Autodesk Fusion 360 part; units mm, degrees
(part 2 of 5)
ref_plane "工作平面7" through (0, 0, 26) normal (0, 0, 1) x (1, 0, 0) in component "L2_RemovableGrate"
sketch "草图7 (6)" plane through (0, 0, 26) normal (0, 0, 1) x (1, 0, 0) in component "L2_RemovableGrate"
  line L0 (299, 60.3) -> (303, 60.3)
  line L1 (303, 60.3) -> (303, 129.7)
  line L2 (303, 129.7) -> (299, 129.7)
  line L3 (299, 129.7) -> (299, 60.3)
  dimension "d537" = 299
  dimension "d539" = 4
  dimension "d540" = 69.4
  constraint horizontal L0
  constraint vertical L1
  constraint horizontal L2
  constraint vertical L3
  measures "d537" horizontal distance of origin L0.start
  measures "d539" horizontal distance of L0.start L0.end
  measures "d540" vertical distance of L0.end L1.end
extrude "Drain slot 6''" cut sketch "草图7 (6)" along normal blind 4 bodies 6 in component "L2_RemovableGrate"
ref_plane "工作平面8" through (0, 0, 26) normal (0, 0, 1) x (1, 0, 0) in component "L2_RemovableGrate"
sketch "草图8 (6)" plane through (0, 0, 26) normal (0, 0, 1) x (1, 0, 0) in component "L2_RemovableGrate"
  line L0 (309, 60.3) -> (313, 60.3)
  line L1 (313, 60.3) -> (313, 129.7)
  line L2 (313, 129.7) -> (309, 129.7)
  line L3 (309, 129.7) -> (309, 60.3)
  dimension "d545" = 309
  dimension "d547" = 4
  dimension "d548" = 69.4
  constraint horizontal L0
  constraint vertical L1
  constraint horizontal L2
  constraint vertical L3
  measures "d545" horizontal distance of origin L0.start
  measures "d547" horizontal distance of L0.start L0.end
  measures "d548" vertical distance of L0.end L1.end
extrude "Drain slot 7''" cut sketch "草图8 (6)" along normal blind 4 bodies 6 in component "L2_RemovableGrate"
ref_plane "工作平面9" through (0, 0, 26) normal (0, 0, 1) x (1, 0, 0) in component "L2_RemovableGrate"
sketch "草图9 (3)" plane through (0, 0, 26) normal (0, 0, 1) x (1, 0, 0) in component "L2_RemovableGrate"
  line L0 (319, 60.3) -> (323, 60.3)
  line L1 (323, 60.3) -> (323, 129.7)
  line L2 (323, 129.7) -> (319, 129.7)
  line L3 (319, 129.7) -> (319, 60.3)
  dimension "d553" = 319
  dimension "d555" = 4
  dimension "d556" = 69.4
  constraint horizontal L0
  constraint vertical L1
  constraint horizontal L2
  constraint vertical L3
  measures "d553" horizontal distance of origin L0.start
  measures "d555" horizontal distance of L0.start L0.end
  measures "d556" vertical distance of L0.end L1.end
extrude "Drain slot 8''" cut sketch "草图9 (3)" along normal blind 4 bodies 6 in component "L2_RemovableGrate"
ref_plane "工作平面10" through (0, 0, 26) normal (0, 0, 1) x (1, 0, 0) in component "L2_RemovableGrate"
sketch "草图10 (3)" plane through (0, 0, 26) normal (0, 0, 1) x (1, 0, 0) in component "L2_RemovableGrate"
  line L0 (329, 60.3) -> (333, 60.3)
  line L1 (333, 60.3) -> (333, 129.7)
  line L2 (333, 129.7) -> (329, 129.7)
  line L3 (329, 129.7) -> (329, 60.3)
  dimension "d561" = 329
  dimension "d563" = 4
  dimension "d564" = 69.4
  constraint horizontal L0
  constraint vertical L1
  constraint horizontal L2
  constraint vertical L3
  measures "d561" horizontal distance of origin L0.start
  measures "d563" horizontal distance of L0.start L0.end
  measures "d564" vertical distance of L0.end L1.end
extrude "Drain slot 9''" cut sketch "草图10 (3)" along normal blind 4 bodies 6 in component "L2_RemovableGrate"
ref_plane "工作平面11" through (0, 0, 26) normal (0, 0, 1) x (1, 0, 0) in component "L2_RemovableGrate"
sketch "草图11 (3)" plane through (0, 0, 26) normal (0, 0, 1) x (1, 0, 0) in component "L2_RemovableGrate"
  line L0 (339, 60.3) -> (343, 60.3)
  line L1 (343, 60.3) -> (343, 129.7)
  line L2 (343, 129.7) -> (339, 129.7)
  line L3 (339, 129.7) -> (339, 60.3)
  dimension "d569" = 339
  dimension "d571" = 4
  dimension "d572" = 69.4
  constraint horizontal L0
  constraint vertical L1
  constraint horizontal L2
  constraint vertical L3
  measures "d569" horizontal distance of origin L0.start
  measures "d571" horizontal distance of L0.start L0.end
  measures "d572" vertical distance of L0.end L1.end
extrude "Drain slot 10''" cut sketch "草图11 (3)" along normal blind 4 bodies 6 in component "L2_RemovableGrate"
ref_plane "工作平面12" through (0, 0, 26) normal (0, 0, 1) x (1, 0, 0) in component "L2_RemovableGrate"
sketch "草图12 (3)" plane through (0, 0, 26) normal (0, 0, 1) x (1, 0, 0) in component "L2_RemovableGrate"
  line L0 (349, 60.3) -> (353, 60.3)
  line L1 (353, 60.3) -> (353, 129.7)
  line L2 (353, 129.7) -> (349, 129.7)
  line L3 (349, 129.7) -> (349, 60.3)
  dimension "d577" = 349
  dimension "d579" = 4
  dimension "d580" = 69.4
  constraint horizontal L0
  constraint vertical L1
  constraint horizontal L2
  constraint vertical L3
  measures "d577" horizontal distance of origin L0.start
  measures "d579" horizontal distance of L0.start L0.end
  measures "d580" vertical distance of L0.end L1.end
extrude "Drain slot 11''" cut sketch "草图12 (3)" along normal blind 4 bodies 6 in component "L2_RemovableGrate"
ref_plane "工作平面13" through (0, 0, 26) normal (0, 0, 1) x (1, 0, 0) in component "L2_RemovableGrate"
sketch "草图13 (3)" plane through (0, 0, 26) normal (0, 0, 1) x (1, 0, 0) in component "L2_RemovableGrate"
  line L0 (359, 60.3) -> (363, 60.3)
  line L1 (363, 60.3) -> (363, 129.7)
  line L2 (363, 129.7) -> (359, 129.7)
  line L3 (359, 129.7) -> (359, 60.3)
  dimension "d585" = 359
  dimension "d587" = 4
  dimension "d588" = 69.4
  constraint horizontal L0
  constraint vertical L1
  constraint horizontal L2
  constraint vertical L3
  measures "d585" horizontal distance of origin L0.start
  measures "d587" horizontal distance of L0.start L0.end
  measures "d588" vertical distance of L0.end L1.end
extrude "Drain slot 12'" cut sketch "草图13 (3)" along normal blind 4 bodies 6 in component "L2_RemovableGrate"
ref_plane "工作平面14" through (0, 0, 26) normal (0, 0, 1) x (1, 0, 0) in component "L2_RemovableGrate"
sketch "草图14 (2)" plane through (0, 0, 26) normal (0, 0, 1) x (1, 0, 0) in component "L2_RemovableGrate"
  line L0 (369, 60.3) -> (373, 60.3)
  line L1 (373, 60.3) -> (373, 129.7)
  line L2 (373, 129.7) -> (369, 129.7)
  line L3 (369, 129.7) -> (369, 60.3)
  dimension "d593" = 369
  dimension "d595" = 4
  dimension "d596" = 69.4
  constraint horizontal L0
  constraint vertical L1
  constraint horizontal L2
  constraint vertical L3
  measures "d593" horizontal distance of origin L0.start
  measures "d595" horizontal distance of L0.start L0.end
  measures "d596" vertical distance of L0.end L1.end
extrude "Drain slot 13'" cut sketch "草图14 (2)" along normal blind 4 bodies 6 in component "L2_RemovableGrate"
ref_plane "工作平面15" through (0, 0, 26) normal (0, 0, 1) x (1, 0, 0) in component "L2_RemovableGrate"
sketch "草图15 (2)" plane through (0, 0, 26) normal (0, 0, 1) x (1, 0, 0) in component "L2_RemovableGrate"
  line L0 (379, 60.3) -> (383, 60.3)
  line L1 (383, 60.3) -> (383, 129.7)
  line L2 (383, 129.7) -> (379, 129.7)
  line L3 (379, 129.7) -> (379, 60.3)
  dimension "d601" = 379
  dimension "d603" = 4
  dimension "d604" = 69.4
  constraint horizontal L0
  constraint vertical L1
  constraint horizontal L2
  constraint vertical L3
  measures "d601" horizontal distance of origin L0.start
  measures "d603" horizontal distance of L0.start L0.end
  measures "d604" vertical distance of L0.end L1.end
extrude "Drain slot 14'" cut sketch "草图15 (2)" along normal blind 4 bodies 6 in component "L2_RemovableGrate"
ref_plane "工作平面16" through (0, 0, 26) normal (0, 0, 1) x (1, 0, 0) in component "L2_RemovableGrate"
sketch "草图16 (2)" plane through (0, 0, 26) normal (0, 0, 1) x (1, 0, 0) in component "L2_RemovableGrate"
  line L0 (389, 60.3) -> (393, 60.3)
  line L1 (393, 60.3) -> (393, 129.7)
  line L2 (393, 129.7) -> (389, 129.7)
  line L3 (389, 129.7) -> (389, 60.3)
  dimension "d609" = 389
  dimension "d611" = 4
  dimension "d612" = 69.4
  constraint horizontal L0
  constraint vertical L1
  constraint horizontal L2
  constraint vertical L3
  measures "d609" horizontal distance of origin L0.start
  measures "d611" horizontal distance of L0.start L0.end
  measures "d612" vertical distance of L0.end L1.end
extrude "Drain slot 15'" cut sketch "草图16 (2)" along normal blind 4 bodies 6 in component "L2_RemovableGrate"
ref_plane "工作平面17" through (0, 0, 26) normal (0, 0, 1) x (1, 0, 0) in component "L2_RemovableGrate"
sketch "草图17 (2)" plane through (0, 0, 26) normal (0, 0, 1) x (1, 0, 0) in component "L2_RemovableGrate"
  line L0 (399, 60.3) -> (403, 60.3)
  line L1 (403, 60.3) -> (403, 129.7)
  line L2 (403, 129.7) -> (399, 129.7)
  line L3 (399, 129.7) -> (399, 60.3)
  dimension "d617" = 399
  dimension "d619" = 4
  dimension "d620" = 69.4
  constraint horizontal L0
  constraint vertical L1
  constraint horizontal L2
  constraint vertical L3
  measures "d617" horizontal distance of origin L0.start
  measures "d619" horizontal distance of L0.start L0.end
  measures "d620" vertical distance of L0.end L1.end
extrude "Drain slot 16" cut sketch "草图17 (2)" along normal blind 4 bodies 6 in component "L2_RemovableGrate"
ref_plane "工作平面18" through (0, 0, 26) normal (0, 0, 1) x (1, 0, 0) in component "L2_RemovableGrate"
sketch "草图18" plane through (0, 0, 26) normal (0, 0, 1) x (1, 0, 0) in component "L2_RemovableGrate"
  line L0 (409, 60.3) -> (413, 60.3)
  line L1 (413, 60.3) -> (413, 129.7)
  line L2 (413, 129.7) -> (409, 129.7)
  line L3 (409, 129.7) -> (409, 60.3)
  dimension "d625" = 409
  dimension "d627" = 4
  dimension "d628" = 69.4
  constraint horizontal L0
  constraint vertical L1
  constraint horizontal L2
  constraint vertical L3
  measures "d625" horizontal distance of origin L0.start
  measures "d627" horizontal distance of L0.start L0.end
  measures "d628" vertical distance of L0.end L1.end
extrude "Drain slot 17" cut sketch "草图18" along normal blind 4 bodies 6 in component "L2_RemovableGrate"
ref_plane "工作平面19" through (0, 0, 26) normal (0, 0, 1) x (1, 0, 0) in component "L2_RemovableGrate"
sketch "草图19" plane through (0, 0, 26) normal (0, 0, 1) x (1, 0, 0) in component "L2_RemovableGrate"
  line L0 (323, 132.7) -> (339, 132.7)
  line L1 (339, 132.7) -> (339, 137.7)
  line L2 (339, 137.7) -> (323, 137.7)
  line L3 (323, 137.7) -> (323, 132.7)
  dimension "d633" = 323
  dimension "d634" = 132.7
  dimension "d635" = 16
  dimension "d636" = 5
  constraint horizontal L0
  constraint vertical L1
  constraint horizontal L2
  constraint vertical L3
  measures "d633" horizontal distance of origin L0.start
  measures "d634" vertical distance of origin L0.start
  measures "d635" horizontal distance of L0.start L0.end
  measures "d636" vertical distance of L0.end L1.end
extrude "Finger lift notch''" cut sketch "草图19" along normal blind 4 bodies 6 in component "L2_RemovableGrate"
chamfer "R03 touch edge chamfer'''''" distance 0.4 angle 45 5 edges at (279.15, 136.7, 30) (235.3, 95, 30) (331, 53.3, 30) (426.7, 95, 30) (382.85, 136.7, 30) on bodies 6 in component "L2_RemovableGrate"
ref_plane "工作平面1" through (0, 0, 10) normal (0, 0, 1) x (1, 0, 0) in component "R2_Integrated"
sketch "草图1 (7)" plane through (0, 0, 10) normal (0, 0, 1) x (1, 0, 0) in component "R2_Integrated"
  line L0 (726, 50) -> (860, 50)
  line L1 (860, 50) -> (860, 140)
  line L2 (860, 140) -> (726, 140)
  line L3 (726, 140) -> (726, 50)
  dimension "d642" = 726
  dimension "d643" = 50
  dimension "d644" = 134
  dimension "d645" = 90
  constraint horizontal L0
  constraint vertical L1
  constraint horizontal L2
  constraint vertical L3
  measures "d642" horizontal distance of origin L0.start
  measures "d643" vertical distance of origin L0.start
  measures "d644" horizontal distance of L0.start L0.end
  measures "d645" vertical distance of L0.end L1.end
extrude "R04 pan blank'''" add sketch "草图1 (7)" along normal blind 20 separate body makes body 7 in component "R2_Integrated"
fillet "Outside corner rounds'''" radius 3 4 edges at (726, 140, 20) (860, 140, 20) (860, 50, 20) (726, 50, 20) on bodies 7 in component "R2_Integrated"
ref_plane "工作平面2" through (729, 0, 0) normal (1, 0, 0) x (0, 1, 0) in component "R2_Integrated"
sketch "草图2 (7)" plane through (729, 0, 0) normal (1, 0, 0) x (0, 0, -1) in component "R2_Integrated"
  line L0 (-22.1441, 53) -> (-13, 140)
  line L1 (-13, 140) -> (-31, 140)
  line L2 (-31, 140) -> (-31, 53)
  line L3 (-31, 53) -> (-22.1441, 53)
  dimension "d654" = 13
  dimension "d656" = 31
  constraint horizontal L1
  constraint vertical L2
  constraint horizontal L3
  measures "d654" horizontal distance of origin L0.end
  measures "d656" horizontal distance of origin L1.end
extrude "R04 continuous slope and open edge'''" cut sketch "草图2 (7)" along normal blind 128 bodies 7 in component "R2_Integrated"
ref_plane "工作平面3" through (0, 0, 10) normal (0, 0, 1) x (1, 0, 0) in component "R2_Integrated"
sketch "草图3 (7)" plane through (0, 0, 10) normal (0, 0, 1) x (1, 0, 0) in component "R2_Integrated"
  line L0 (729, 53) -> (741, 53)
  line L1 (741, 53) -> (741, 65)
  line L2 (741, 65) -> (729, 65)
  line L3 (729, 65) -> (729, 53)
  dimension "d661" = 729
  dimension "d663" = 12
  dimension "d664" = 12
  constraint horizontal L0
  constraint vertical L1
  constraint horizontal L2
  constraint vertical L3
  measures "d661" horizontal distance of origin L0.start
  measures "d663" horizontal distance of L0.start L0.end
  measures "d664" vertical distance of L0.end L1.end
extrude "Grate seat 00'''" add sketch "草图3 (7)" along normal blind 16 bodies 7 in component "R2_Integrated"
ref_plane "工作平面4" through (0, 0, 10) normal (0, 0, 1) x (1, 0, 0) in component "R2_Integrated"
sketch "草图4 (7)" plane through (0, 0, 10) normal (0, 0, 1) x (1, 0, 0) in component "R2_Integrated"
  line L0 (729, 125) -> (741, 125)
  line L1 (741, 125) -> (741, 137)
  line L2 (741, 137) -> (729, 137)
  line L3 (729, 137) -> (729, 125)
  dimension "d669" = 729
  dimension "d670" = 125
  dimension "d671" = 12
  dimension "d672" = 12
  constraint horizontal L0
  constraint vertical L1
  constraint horizontal L2
  constraint vertical L3
  measures "d669" horizontal distance of origin L0.start
  measures "d670" vertical distance of origin L0.start
  measures "d671" horizontal distance of L0.start L0.end
  measures "d672" vertical distance of L0.end L1.end
extrude "Grate seat 01'''" add sketch "草图4 (7)" along normal blind 16 bodies 7 in component "R2_Integrated"
ref_plane "工作平面5" through (0, 0, 10) normal (0, 0, 1) x (1, 0, 0) in component "R2_Integrated"
sketch "草图5 (7)" plane through (0, 0, 10) normal (0, 0, 1) x (1, 0, 0) in component "R2_Integrated"
  line L0 (845, 53) -> (857, 53)
  line L1 (857, 53) -> (857, 65)
  line L2 (857, 65) -> (845, 65)
  line L3 (845, 65) -> (845, 53)
  dimension "d677" = 845
  dimension "d679" = 12
  dimension "d680" = 12
  constraint horizontal L0
  constraint vertical L1
  constraint horizontal L2
  constraint vertical L3
  measures "d677" horizontal distance of origin L0.start
  measures "d679" horizontal distance of L0.start L0.end
  measures "d680" vertical distance of L0.end L1.end
extrude "Grate seat 10'''" add sketch "草图5 (7)" along normal blind 16 bodies 7 in component "R2_Integrated"
ref_plane "工作平面6" through (0, 0, 10) normal (0, 0, 1) x (1, 0, 0) in component "R2_Integrated"
sketch "草图6 (7)" plane through (0, 0, 10) normal (0, 0, 1) x (1, 0, 0) in component "R2_Integrated"
  line L0 (845, 125) -> (857, 125)
  line L1 (857, 125) -> (857, 137)
  line L2 (857, 137) -> (845, 137)
  line L3 (845, 137) -> (845, 125)
  dimension "d685" = 845
  dimension "d686" = 125
  dimension "d687" = 12
  dimension "d688" = 12
  constraint horizontal L0
  constraint vertical L1
  constraint horizontal L2
  constraint vertical L3
  measures "d685" horizontal distance of origin L0.start
  measures "d686" vertical distance of origin L0.start
  measures "d687" horizontal distance of L0.start L0.end
  measures "d688" vertical distance of L0.end L1.end
extrude "Grate seat 11'''" add sketch "草图6 (7)" along normal blind 16 bodies 7 in component "R2_Integrated"
ref_plane "工作平面7" through (0, 0, 0) normal (0, 0, 1) x (1, 0, 0) in component "R2_Integrated"
sketch "草图7 (7)" plane through (0, 0, 0) normal (0, 0, 1) x (1, 0, 0) in component "R2_Integrated"
  line L0 (729, 50) -> (737, 50)
  line L1 (737, 50) -> (737, 131)
  line L2 (737, 131) -> (729, 131)
  line L3 (729, 131) -> (729, 50)
  dimension "d693" = 729
  dimension "d694" = 50
  dimension "d695" = 8
  dimension "d696" = 81
  constraint horizontal L0
  constraint vertical L1
  constraint horizontal L2
  constraint vertical L3
  measures "d693" horizontal distance of origin L0.start
  measures "d694" vertical distance of origin L0.start
  measures "d695" horizontal distance of L0.start L0.end
  measures "d696" vertical distance of L0.end L1.end
extrude "R04 low integral runner 0'''" add sketch "草图7 (7)" along normal blind 10 bodies 7 in component "R2_Integrated"
ref_plane "工作平面8" through (0, 0, 0) normal (0, 0, 1) x (1, 0, 0) in component "R2_Integrated"
sketch "草图8 (7)" plane through (0, 0, 0) normal (0, 0, 1) x (1, 0, 0) in component "R2_Integrated"
  line L0 (849, 50) -> (857, 50)
  line L1 (857, 50) -> (857, 131)
  line L2 (857, 131) -> (849, 131)
  line L3 (849, 131) -> (849, 50)
  dimension "d701" = 849
  dimension "d702" = 50
  dimension "d703" = 8
  dimension "d704" = 81
  constraint horizontal L0
  constraint vertical L1
  constraint horizontal L2
  constraint vertical L3
  measures "d701" horizontal distance of origin L0.start
  measures "d702" vertical distance of origin L0.start
  measures "d703" horizontal distance of L0.start L0.end
  measures "d704" vertical distance of L0.end L1.end
extrude "R04 low integral runner 1'''" add sketch "草图8 (7)" along normal blind 10 bodies 7 in component "R2_Integrated"
chamfer "R03 touch edge chamfer''''''" distance 0.4 angle 45 5 edges at (793, 53, 30) (729, 96.5, 30) (857, 96.5, 30) (726, 95, 30) (860, 95, 30) on bodies 7 in component "R2_Integrated"
ref_plane "工作平面1" through (0, 0, 26) normal (0, 0, 1) x (1, 0, 0) in component "R2_RemovableGrate"
sketch "草图1 (8)" plane through (0, 0, 26) normal (0, 0, 1) x (1, 0, 0) in component "R2_RemovableGrate"
  line L0 (729.3, 53.3) -> (856.7, 53.3)
  line L1 (856.7, 53.3) -> (856.7, 136.7)
  line L2 (856.7, 136.7) -> (729.3, 136.7)
  line L3 (729.3, 136.7) -> (729.3, 53.3)
  dimension "d710" = 729.3
  dimension "d712" = 127.4
  dimension "d713" = 83.4
  constraint horizontal L0
  constraint vertical L1
  constraint horizontal L2
  constraint vertical L3
  measures "d710" horizontal distance of origin L0.start
  measures "d712" horizontal distance of L0.start L0.end
  measures "d713" vertical distance of L0.end L1.end
extrude "Horizontal removable deck'''" add sketch "草图1 (8)" along normal blind 4 separate body makes body 8 in component "R2_RemovableGrate"
ref_plane "工作平面2" through (0, 0, 26) normal (0, 0, 1) x (1, 0, 0) in component "R2_RemovableGrate"
sketch "草图2 (8)" plane through (0, 0, 26) normal (0, 0, 1) x (1, 0, 0) in component "R2_RemovableGrate"
  line L0 (741, 60.3) -> (745, 60.3)
  line L1 (745, 60.3) -> (745, 129.7)
  line L2 (745, 129.7) -> (741, 129.7)
  line L3 (741, 129.7) -> (741, 60.3)
  dimension "d718" = 741
  dimension "d720" = 4
  dimension "d721" = 69.4
  constraint horizontal L0
  constraint vertical L1
  constraint horizontal L2
  constraint vertical L3
  measures "d718" horizontal distance of origin L0.start
  measures "d720" horizontal distance of L0.start L0.end
  measures "d721" vertical distance of L0.end L1.end
extrude "Drain slot 1'''" cut sketch "草图2 (8)" along normal blind 4 bodies 8 in component "R2_RemovableGrate"
ref_plane "工作平面3" through (0, 0, 26) normal (0, 0, 1) x (1, 0, 0) in component "R2_RemovableGrate"
sketch "草图3 (8)" plane through (0, 0, 26) normal (0, 0, 1) x (1, 0, 0) in component "R2_RemovableGrate"
  line L0 (751, 60.3) -> (755, 60.3)
  line L1 (755, 60.3) -> (755, 129.7)
  line L2 (755, 129.7) -> (751, 129.7)
  line L3 (751, 129.7) -> (751, 60.3)
  dimension "d726" = 751
  dimension "d728" = 4
  dimension "d729" = 69.4
  constraint horizontal L0
  constraint vertical L1
  constraint horizontal L2
  constraint vertical L3
  measures "d726" horizontal distance of origin L0.start
  measures "d728" horizontal distance of L0.start L0.end
  measures "d729" vertical distance of L0.end L1.end
extrude "Drain slot 2'''" cut sketch "草图3 (8)" along normal blind 4 bodies 8 in component "R2_RemovableGrate"
ref_plane "工作平面4" through (0, 0, 26) normal (0, 0, 1) x (1, 0, 0) in component "R2_RemovableGrate"
sketch "草图4 (8)" plane through (0, 0, 26) normal (0, 0, 1) x (1, 0, 0) in component "R2_RemovableGrate"
  line L0 (761, 60.3) -> (765, 60.3)
  line L1 (765, 60.3) -> (765, 129.7)
  line L2 (765, 129.7) -> (761, 129.7)
  line L3 (761, 129.7) -> (761, 60.3)
  dimension "d734" = 761
  dimension "d736" = 4
  dimension "d737" = 69.4
  constraint horizontal L0
  constraint vertical L1
  constraint horizontal L2
  constraint vertical L3
  measures "d734" horizontal distance of origin L0.start
  measures "d736" horizontal distance of L0.start L0.end
  measures "d737" vertical distance of L0.end L1.end
extrude "Drain slot 3'''" cut sketch "草图4 (8)" along normal blind 4 bodies 8 in component "R2_RemovableGrate"
ref_plane "工作平面5" through (0, 0, 26) normal (0, 0, 1) x (1, 0, 0) in component "R2_RemovableGrate"
sketch "草图5 (8)" plane through (0, 0, 26) normal (0, 0, 1) x (1, 0, 0) in component "R2_RemovableGrate"
  line L0 (771, 60.3) -> (775, 60.3)
  line L1 (775, 60.3) -> (775, 129.7)
  line L2 (775, 129.7) -> (771, 129.7)
  line L3 (771, 129.7) -> (771, 60.3)
  dimension "d742" = 771
  dimension "d744" = 4
  dimension "d745" = 69.4
  constraint horizontal L0
  constraint vertical L1
  constraint horizontal L2
  constraint vertical L3
  measures "d742" horizontal distance of origin L0.start
  measures "d744" horizontal distance of L0.start L0.end
  measures "d745" vertical distance of L0.end L1.end
extrude "Drain slot 4'''" cut sketch "草图5 (8)" along normal blind 4 bodies 8 in component "R2_RemovableGrate"
ref_plane "工作平面6" through (0, 0, 26) normal (0, 0, 1) x (1, 0, 0) in component "R2_RemovableGrate"
sketch "草图6 (8)" plane through (0, 0, 26) normal (0, 0, 1) x (1, 0, 0) in component "R2_RemovableGrate"
  line L0 (781, 60.3) -> (785, 60.3)
  line L1 (785, 60.3) -> (785, 129.7)
  line L2 (785, 129.7) -> (781, 129.7)
  line L3 (781, 129.7) -> (781, 60.3)
  dimension "d750" = 781
  dimension "d752" = 4
  dimension "d753" = 69.4
  constraint horizontal L0
  constraint vertical L1
  constraint horizontal L2
  constraint vertical L3
  measures "d750" horizontal distance of origin L0.start
  measures "d752" horizontal distance of L0.start L0.end
  measures "d753" vertical distance of L0.end L1.end
extrude "Drain slot 5'''" cut sketch "草图6 (8)" along normal blind 4 bodies 8 in component "R2_RemovableGrate"
ref_plane "工作平面7" through (0, 0, 26) normal (0, 0, 1) x (1, 0, 0) in component "R2_RemovableGrate"
sketch "草图7 (8)" plane through (0, 0, 26) normal (0, 0, 1) x (1, 0, 0) in component "R2_RemovableGrate"
  line L0 (791, 60.3) -> (795, 60.3)
  line L1 (795, 60.3) -> (795, 129.7)
  line L2 (795, 129.7) -> (791, 129.7)
  line L3 (791, 129.7) -> (791, 60.3)
  dimension "d758" = 791
  dimension "d760" = 4
  dimension "d761" = 69.4
  constraint horizontal L0
  constraint vertical L1
  constraint horizontal L2
  constraint vertical L3
  measures "d758" horizontal distance of origin L0.start
  measures "d760" horizontal distance of L0.start L0.end
  measures "d761" vertical distance of L0.end L1.end
extrude "Drain slot 6'''" cut sketch "草图7 (8)" along normal blind 4 bodies 8 in component "R2_RemovableGrate"
ref_plane "工作平面8" through (0, 0, 26) normal (0, 0, 1) x (1, 0, 0) in component "R2_RemovableGrate"
sketch "草图8 (8)" plane through (0, 0, 26) normal (0, 0, 1) x (1, 0, 0) in component "R2_RemovableGrate"
  line L0 (801, 60.3) -> (805, 60.3)
  line L1 (805, 60.3) -> (805, 129.7)
  line L2 (805, 129.7) -> (801, 129.7)
  line L3 (801, 129.7) -> (801, 60.3)
  dimension "d766" = 801
  dimension "d768" = 4
  dimension "d769" = 69.4
  constraint horizontal L0
  constraint vertical L1
  constraint horizontal L2
  constraint vertical L3
  measures "d766" horizontal distance of origin L0.start
  measures "d768" horizontal distance of L0.start L0.end
  measures "d769" vertical distance of L0.end L1.end
extrude "Drain slot 7'''" cut sketch "草图8 (8)" along normal blind 4 bodies 8 in component "R2_RemovableGrate"
ref_plane "工作平面9" through (0, 0, 26) normal (0, 0, 1) x (1, 0, 0) in component "R2_RemovableGrate"
sketch "草图9 (4)" plane through (0, 0, 26) normal (0, 0, 1) x (1, 0, 0) in component "R2_RemovableGrate"
  line L0 (811, 60.3) -> (815, 60.3)
  line L1 (815, 60.3) -> (815, 129.7)
  line L2 (815, 129.7) -> (811, 129.7)
  line L3 (811, 129.7) -> (811, 60.3)
  dimension "d774" = 811
  dimension "d776" = 4
  dimension "d777" = 69.4
  constraint horizontal L0
  constraint vertical L1
  constraint horizontal L2
  constraint vertical L3
  measures "d774" horizontal distance of origin L0.start
  measures "d776" horizontal distance of L0.start L0.end
  measures "d777" vertical distance of L0.end L1.end
extrude "Drain slot 8'''" cut sketch "草图9 (4)" along normal blind 4 bodies 8 in component "R2_RemovableGrate"
ref_plane "工作平面10" through (0, 0, 26) normal (0, 0, 1) x (1, 0, 0) in component "R2_RemovableGrate"
sketch "草图10 (4)" plane through (0, 0, 26) normal (0, 0, 1) x (1, 0, 0) in component "R2_RemovableGrate"
  line L0 (821, 60.3) -> (825, 60.3)
  line L1 (825, 60.3) -> (825, 129.7)
  line L2 (825, 129.7) -> (821, 129.7)
  line L3 (821, 129.7) -> (821, 60.3)
  dimension "d782" = 821
  dimension "d784" = 4
  dimension "d785" = 69.4
  constraint horizontal L0
  constraint vertical L1
  constraint horizontal L2
  constraint vertical L3
  measures "d782" horizontal distance of origin L0.start
  measures "d784" horizontal distance of L0.start L0.end
  measures "d785" vertical distance of L0.end L1.end
extrude "Drain slot 9'''" cut sketch "草图10 (4)" along normal blind 4 bodies 8 in component "R2_RemovableGrate"
ref_plane "工作平面11" through (0, 0, 26) normal (0, 0, 1) x (1, 0, 0) in component "R2_RemovableGrate"
sketch "草图11 (4)" plane through (0, 0, 26) normal (0, 0, 1) x (1, 0, 0) in component "R2_RemovableGrate"
  line L0 (831, 60.3) -> (835, 60.3)
  line L1 (835, 60.3) -> (835, 129.7)
  line L2 (835, 129.7) -> (831, 129.7)
  line L3 (831, 129.7) -> (831, 60.3)
  dimension "d790" = 831
  dimension "d792" = 4
  dimension "d793" = 69.4
  constraint horizontal L0
  constraint vertical L1
  constraint horizontal L2
  constraint vertical L3
  measures "d790" horizontal distance of origin L0.start
  measures "d792" horizontal distance of L0.start L0.end
  measures "d793" vertical distance of L0.end L1.end
extrude "Drain slot 10'''" cut sketch "草图11 (4)" along normal blind 4 bodies 8 in component "R2_RemovableGrate"
ref_plane "工作平面12" through (0, 0, 26) normal (0, 0, 1) x (1, 0, 0) in component "R2_RemovableGrate"
sketch "草图12 (4)" plane through (0, 0, 26) normal (0, 0, 1) x (1, 0, 0) in component "R2_RemovableGrate"
  line L0 (841, 60.3) -> (845, 60.3)
  line L1 (845, 60.3) -> (845, 129.7)
  line L2 (845, 129.7) -> (841, 129.7)
  line L3 (841, 129.7) -> (841, 60.3)
  dimension "d798" = 841
  dimension "d800" = 4
  dimension "d801" = 69.4
  constraint horizontal L0
  constraint vertical L1
  constraint horizontal L2
  constraint vertical L3
  measures "d798" horizontal distance of origin L0.start
  measures "d800" horizontal distance of L0.start L0.end
  measures "d801" vertical distance of L0.end L1.end
extrude "Drain slot 11'''" cut sketch "草图12 (4)" along normal blind 4 bodies 8 in component "R2_RemovableGrate"
ref_plane "工作平面13" through (0, 0, 26) normal (0, 0, 1) x (1, 0, 0) in component "R2_RemovableGrate"
sketch "草图13 (4)" plane through (0, 0, 26) normal (0, 0, 1) x (1, 0, 0) in component "R2_RemovableGrate"
  line L0 (785, 132.7) -> (801, 132.7)
  line L1 (801, 132.7) -> (801, 137.7)
  line L2 (801, 137.7) -> (785, 137.7)
  line L3 (785, 137.7) -> (785, 132.7)
  dimension "d806" = 785
  dimension "d807" = 132.7
  dimension "d808" = 16
  dimension "d809" = 5
  constraint horizontal L0
  constraint vertical L1
  constraint horizontal L2
  constraint vertical L3
  measures "d806" horizontal distance of origin L0.start
  measures "d807" vertical distance of origin L0.start
  measures "d808" horizontal distance of L0.start L0.end
  measures "d809" vertical distance of L0.end L1.end
extrude "Finger lift notch'''" cut sketch "草图13 (4)" along normal blind 4 bodies 8 in component "R2_RemovableGrate"
chamfer "R03 touch edge chamfer'''''''" distance 0.4 angle 45 5 edges at (757.15, 136.7, 30) (729.3, 95, 30) (793, 53.3, 30) (856.7, 95, 30) (828.85, 136.7, 30) on bodies 8 in component "R2_RemovableGrate"
ref_plane "工作平面1" through (0, 0, 10) normal (0, 0, 1) x (1, 0, 0) in component "LS_Integrated"
sketch "草图1 (9)" plane through (0, 0, 10) normal (0, 0, 1) x (1, 0, 0) in component "LS_Integrated"
  line L0 (50, 142) -> (170, 142)
  line L1 (170, 142) -> (170, 322)
  line L2 (170, 322) -> (50, 322)
  line L3 (50, 322) -> (50, 142)
  dimension "d815" = 50
  dimension "d816" = 142
  dimension "d817" = 120
  dimension "d818" = 180
  constraint horizontal L0
  constraint vertical L1
  constraint horizontal L2
  constraint vertical L3
  measures "d815" horizontal distance of origin L0.start
  measures "d816" vertical distance of origin L0.start
  measures "d817" horizontal distance of L0.start L0.end
  measures "d818" vertical distance of L0.end L1.end
extrude "R04 pan blank''''" add sketch "草图1 (9)" along normal blind 20 separate body makes body 9 in component "LS_Integrated"
fillet "Outside corner rounds''''" radius 3 4 edges at (50, 322, 20) (170, 322, 20) (170, 142, 20) (50, 142, 20) on bodies 9 in component "LS_Integrated"
ref_plane "工作平面2" through (0, 319, 0) normal (0, 1, 0) x (0, 0, 1) in component "LS_Integrated"
sketch "草图2 (9)" plane through (0, 319, 0) normal (0, 1, 0) x (1, 0, 0) in component "LS_Integrated"
  line L0 (53, -25.2972) -> (170, -13)
  line L1 (170, -13) -> (170, -31)
  line L2 (170, -31) -> (53, -31)
  line L3 (53, -31) -> (53, -25.2972)
  dimension "d826" = 25.2972
  dimension "d828" = 13
  dimension "d829" = 31
  constraint vertical L1
  constraint horizontal L2
  constraint vertical L3
  measures "d826" vertical distance of origin L0.start
  measures "d828" vertical distance of origin L0.end
  measures "d829" vertical distance of origin L1.end
extrude "R04 continuous slope and open edge''''" cut sketch "草图2 (9)" against normal blind 174 bodies 9 in component "LS_Integrated"
ref_plane "工作平面3" through (0, 0, 10) normal (0, 0, 1) x (1, 0, 0) in component "LS_Integrated"
sketch "草图3 (9)" plane through (0, 0, 10) normal (0, 0, 1) x (1, 0, 0) in component "LS_Integrated"
  line L0 (53, 307) -> (65, 307)
  line L1 (65, 307) -> (65, 319)
  line L2 (65, 319) -> (53, 319)
  line L3 (53, 319) -> (53, 307)
  dimension "d835" = 307
  dimension "d836" = 12
  dimension "d837" = 12
  constraint horizontal L0
  constraint vertical L1
  constraint horizontal L2
  constraint vertical L3
  measures "d835" vertical distance of origin L0.start
  measures "d836" horizontal distance of L0.start L0.end
  measures "d837" vertical distance of L0.end L1.end
extrude "Grate seat 00''''" add sketch "草图3 (9)" along normal blind 16 bodies 9 in component "LS_Integrated"
ref_plane "工作平面4" through (0, 0, 10) normal (0, 0, 1) x (1, 0, 0) in component "LS_Integrated"
sketch "草图4 (9)" plane through (0, 0, 10) normal (0, 0, 1) x (1, 0, 0) in component "LS_Integrated"
  line L0 (155, 307) -> (167, 307)
  line L1 (167, 307) -> (167, 319)
  line L2 (167, 319) -> (155, 319)
  line L3 (155, 319) -> (155, 307)
  dimension "d842" = 155
  dimension "d843" = 307
  dimension "d844" = 12
  dimension "d845" = 12
  constraint horizontal L0
  constraint vertical L1
  constraint horizontal L2
  constraint vertical L3
  measures "d842" horizontal distance of origin L0.start
  measures "d843" vertical distance of origin L0.start
  measures "d844" horizontal distance of L0.start L0.end
  measures "d845" vertical distance of L0.end L1.end
extrude "Grate seat 01''''" add sketch "草图4 (9)" along normal blind 16 bodies 9 in component "LS_Integrated"
ref_plane "工作平面5" through (0, 0, 10) normal (0, 0, 1) x (1, 0, 0) in component "LS_Integrated"
sketch "草图5 (9)" plane through (0, 0, 10) normal (0, 0, 1) x (1, 0, 0) in component "LS_Integrated"
  line L0 (53, 145) -> (65, 145)
  line L1 (65, 145) -> (65, 157)
  line L2 (65, 157) -> (53, 157)
  line L3 (53, 157) -> (53, 145)
  dimension "d851" = 145
  dimension "d852" = 12
  dimension "d853" = 12
  constraint horizontal L0
  constraint vertical L1
  constraint horizontal L2
  constraint vertical L3
  measures "d851" vertical distance of origin L0.start
  measures "d852" horizontal distance of L0.start L0.end
  measures "d853" vertical distance of L0.end L1.end
extrude "Grate seat 10''''" add sketch "草图5 (9)" along normal blind 16 bodies 9 in component "LS_Integrated"
ref_plane "工作平面6" through (0, 0, 10) normal (0, 0, 1) x (1, 0, 0) in component "LS_Integrated"
sketch "草图6 (9)" plane through (0, 0, 10) normal (0, 0, 1) x (1, 0, 0) in component "LS_Integrated"
  line L0 (155, 145) -> (167, 145)
  line L1 (167, 145) -> (167, 157)
  line L2 (167, 157) -> (155, 157)
  line L3 (155, 157) -> (155, 145)
  dimension "d858" = 155
  dimension "d859" = 145
  dimension "d860" = 12
  dimension "d861" = 12
  constraint horizontal L0
  constraint vertical L1
  constraint horizontal L2
  constraint vertical L3
  measures "d858" horizontal distance of origin L0.start
  measures "d859" vertical distance of origin L0.start
  measures "d860" horizontal distance of L0.start L0.end
  measures "d861" vertical distance of L0.end L1.end
extrude "Grate seat 11''''" add sketch "草图6 (9)" along normal blind 16 bodies 9 in component "LS_Integrated"
ref_plane "工作平面7" through (0, 0, 0) normal (0, 0, 1) x (1, 0, 0) in component "LS_Integrated"
sketch "草图7 (9)" plane through (0, 0, 0) normal (0, 0, 1) x (1, 0, 0) in component "LS_Integrated"
  line L0 (50, 311) -> (161, 311)
  line L1 (161, 311) -> (161, 319)
  line L2 (161, 319) -> (50, 319)
  line L3 (50, 319) -> (50, 311)
  dimension "d866" = 50
  dimension "d867" = 311
  dimension "d868" = 111
  dimension "d869" = 8
  constraint horizontal L0
  constraint vertical L1
  constraint horizontal L2
  constraint vertical L3
  measures "d866" horizontal distance of origin L0.start
  measures "d867" vertical distance of origin L0.start
  measures "d868" horizontal distance of L0.start L0.end
  measures "d869" vertical distance of L0.end L1.end
extrude "R04 low integral runner 0''''" add sketch "草图7 (9)" along normal blind 10 bodies 9 in component "LS_Integrated"
ref_plane "工作平面8" through (0, 0, 0) normal (0, 0, 1) x (1, 0, 0) in component "LS_Integrated"
sketch "草图8 (9)" plane through (0, 0, 0) normal (0, 0, 1) x (1, 0, 0) in component "LS_Integrated"
  line L0 (50, 145) -> (161, 145)
  line L1 (161, 145) -> (161, 153)
  line L2 (161, 153) -> (50, 153)
  line L3 (50, 153) -> (50, 145)
  dimension "d874" = 50
  dimension "d875" = 145
  dimension "d876" = 111
  dimension "d877" = 8
  constraint horizontal L0
  constraint vertical L1
  constraint horizontal L2
  constraint vertical L3
  measures "d874" horizontal distance of origin L0.start
  measures "d875" vertical distance of origin L0.start
  measures "d876" horizontal distance of L0.start L0.end
  measures "d877" vertical distance of L0.end L1.end
extrude "R04 low integral runner 1''''" add sketch "草图8 (9)" along normal blind 10 bodies 9 in component "LS_Integrated"
chamfer "R03 touch edge chamfer''''''''" distance 0.4 angle 45 5 edges at (111.5, 145, 30) (53, 232, 30) (111.5, 319, 30) (110, 322, 30) (110, 142, 30) on bodies 9 in component "LS_Integrated"
ref_plane "工作平面1" through (0, 0, 26) normal (0, 0, 1) x (1, 0, 0) in component "LS_RemovableGrate"
sketch "草图1 (10)" plane through (0, 0, 26) normal (0, 0, 1) x (1, 0, 0) in component "LS_RemovableGrate"
  line L0 (53.3, 145.3) -> (166.7, 145.3)
  line L1 (166.7, 145.3) -> (166.7, 318.7)
  line L2 (166.7, 318.7) -> (53.3, 318.7)
  line L3 (53.3, 318.7) -> (53.3, 145.3)
  dimension "d884" = 145.3
  dimension "d885" = 113.4
  dimension "d886" = 173.4
  constraint horizontal L0
  constraint vertical L1
  constraint horizontal L2
  constraint vertical L3
  measures "d884" vertical distance of origin L0.start
  measures "d885" horizontal distance of L0.start L0.end
  measures "d886" vertical distance of L0.end L1.end
extrude "Horizontal removable deck''''" add sketch "草图1 (10)" along normal blind 4 separate body makes body 10 in component "LS_RemovableGrate"
ref_plane "工作平面2" through (0, 0, 26) normal (0, 0, 1) x (1, 0, 0) in component "LS_RemovableGrate"
sketch "草图2 (10)" plane through (0, 0, 26) normal (0, 0, 1) x (1, 0, 0) in component "LS_RemovableGrate"
  line L0 (60.3, 300) -> (159.7, 300)
  line L1 (159.7, 300) -> (159.7, 304)
  line L2 (159.7, 304) -> (60.3, 304)
  line L3 (60.3, 304) -> (60.3, 300)
  dimension "d892" = 300
  dimension "d893" = 99.4
  dimension "d894" = 4
  constraint horizontal L0
  constraint vertical L1
  constraint horizontal L2
  constraint vertical L3
  measures "d892" vertical distance of origin L0.start
  measures "d893" horizontal distance of L0.start L0.end
  measures "d894" vertical distance of L0.end L1.end
extrude "Drain slot 1''''" cut sketch "草图2 (10)" along normal blind 4 bodies 10 in component "LS_RemovableGrate"
ref_plane "工作平面3" through (0, 0, 26) normal (0, 0, 1) x (1, 0, 0) in component "LS_RemovableGrate"
sketch "草图3 (10)" plane through (0, 0, 26) normal (0, 0, 1) x (1, 0, 0) in component "LS_RemovableGrate"
  line L0 (60.3, 290) -> (159.7, 290)
  line L1 (159.7, 290) -> (159.7, 294)
  line L2 (159.7, 294) -> (60.3, 294)
  line L3 (60.3, 294) -> (60.3, 290)
  dimension "d900" = 290
  dimension "d901" = 99.4
  dimension "d902" = 4
  constraint horizontal L0
  constraint vertical L1
  constraint horizontal L2
  constraint vertical L3
  measures "d900" vertical distance of origin L0.start
  measures "d901" horizontal distance of L0.start L0.end
  measures "d902" vertical distance of L0.end L1.end
extrude "Drain slot 2''''" cut sketch "草图3 (10)" along normal blind 4 bodies 10 in component "LS_RemovableGrate"
ref_plane "工作平面4" through (0, 0, 26) normal (0, 0, 1) x (1, 0, 0) in component "LS_RemovableGrate"
sketch "草图4 (10)" plane through (0, 0, 26) normal (0, 0, 1) x (1, 0, 0) in component "LS_RemovableGrate"
  line L0 (60.3, 280) -> (159.7, 280)
  line L1 (159.7, 280) -> (159.7, 284)
  line L2 (159.7, 284) -> (60.3, 284)
  line L3 (60.3, 284) -> (60.3, 280)
  dimension "d908" = 280
  dimension "d909" = 99.4
  dimension "d910" = 4
  constraint horizontal L0
  constraint vertical L1
  constraint horizontal L2
  constraint vertical L3
  measures "d908" vertical distance of origin L0.start
  measures "d909" horizontal distance of L0.start L0.end
  measures "d910" vertical distance of L0.end L1.end
extrude "Drain slot 3''''" cut sketch "草图4 (10)" along normal blind 4 bodies 10 in component "LS_RemovableGrate"
ref_plane "工作平面5" through (0, 0, 26) normal (0, 0, 1) x (1, 0, 0) in component "LS_RemovableGrate"
sketch "草图5 (10)" plane through (0, 0, 26) normal (0, 0, 1) x (1, 0, 0) in component "LS_RemovableGrate"
  line L0 (60.3, 270) -> (159.7, 270)
  line L1 (159.7, 270) -> (159.7, 274)
  line L2 (159.7, 274) -> (60.3, 274)
  line L3 (60.3, 274) -> (60.3, 270)
  dimension "d916" = 270
  dimension "d917" = 99.4
  dimension "d918" = 4
  constraint horizontal L0
  constraint vertical L1
  constraint horizontal L2
  constraint vertical L3
  measures "d916" vertical distance of origin L0.start
  measures "d917" horizontal distance of L0.start L0.end
  measures "d918" vertical distance of L0.end L1.end
extrude "Drain slot 4''''" cut sketch "草图5 (10)" along normal blind 4 bodies 10 in component "LS_RemovableGrate"
ref_plane "工作平面6" through (0, 0, 26) normal (0, 0, 1) x (1, 0, 0) in component "LS_RemovableGrate"
sketch "草图6 (10)" plane through (0, 0, 26) normal (0, 0, 1) x (1, 0, 0) in component "LS_RemovableGrate"
  line L0 (60.3, 260) -> (159.7, 260)
  line L1 (159.7, 260) -> (159.7, 264)
  line L2 (159.7, 264) -> (60.3, 264)
  line L3 (60.3, 264) -> (60.3, 260)
  dimension "d924" = 260
  dimension "d925" = 99.4
  dimension "d926" = 4
  constraint horizontal L0
  constraint vertical L1
  constraint horizontal L2
  constraint vertical L3
  measures "d924" vertical distance of origin L0.start
  measures "d925" horizontal distance of L0.start L0.end
  measures "d926" vertical distance of L0.end L1.end
extrude "Drain slot 5''''" cut sketch "草图6 (10)" along normal blind 4 bodies 10 in component "LS_RemovableGrate"
ref_plane "工作平面7" through (0, 0, 26) normal (0, 0, 1) x (1, 0, 0) in component "LS_RemovableGrate"
sketch "草图7 (10)" plane through (0, 0, 26) normal (0, 0, 1) x (1, 0, 0) in component "LS_RemovableGrate"
  line L0 (60.3, 250) -> (159.7, 250)
  line L1 (159.7, 250) -> (159.7, 254)
  line L2 (159.7, 254) -> (60.3, 254)
  line L3 (60.3, 254) -> (60.3, 250)
  dimension "d932" = 250
  dimension "d933" = 99.4
  dimension "d934" = 4
  constraint horizontal L0
  constraint vertical L1
  constraint horizontal L2
  constraint vertical L3
  measures "d932" vertical distance of origin L0.start
  measures "d933" horizontal distance of L0.start L0.end
  measures "d934" vertical distance of L0.end L1.end
extrude "Drain slot 6''''" cut sketch "草图7 (10)" along normal blind 4 bodies 10 in component "LS_RemovableGrate"
ref_plane "工作平面8" through (0, 0, 26) normal (0, 0, 1) x (1, 0, 0) in component "LS_RemovableGrate"
sketch "草图8 (10)" plane through (0, 0, 26) normal (0, 0, 1) x (1, 0, 0) in component "LS_RemovableGrate"
  line L0 (60.3, 240) -> (159.7, 240)
  line L1 (159.7, 240) -> (159.7, 244)
  line L2 (159.7, 244) -> (60.3, 244)
  line L3 (60.3, 244) -> (60.3, 240)
  dimension "d940" = 240
  dimension "d941" = 99.4
  dimension "d942" = 4
  constraint horizontal L0
  constraint vertical L1
  constraint horizontal L2
  constraint vertical L3
  measures "d940" vertical distance of origin L0.start
  measures "d941" horizontal distance of L0.start L0.end
  measures "d942" vertical distance of L0.end L1.end
extrude "Drain slot 7''''" cut sketch "草图8 (10)" along normal blind 4 bodies 10 in component "LS_RemovableGrate"
ref_plane "工作平面9" through (0, 0, 26) normal (0, 0, 1) x (1, 0, 0) in component "LS_RemovableGrate"
sketch "草图9 (5)" plane through (0, 0, 26) normal (0, 0, 1) x (1, 0, 0) in component "LS_RemovableGrate"
  line L0 (60.3, 230) -> (159.7, 230)
  line L1 (159.7, 230) -> (159.7, 234)
  line L2 (159.7, 234) -> (60.3, 234)
  line L3 (60.3, 234) -> (60.3, 230)
  dimension "d948" = 230
  dimension "d949" = 99.4
  dimension "d950" = 4
  constraint horizontal L0
  constraint vertical L1
  constraint horizontal L2
  constraint vertical L3
  measures "d948" vertical distance of origin L0.start
  measures "d949" horizontal distance of L0.start L0.end
  measures "d950" vertical distance of L0.end L1.end
extrude "Drain slot 8''''" cut sketch "草图9 (5)" along normal blind 4 bodies 10 in component "LS_RemovableGrate"
ref_plane "工作平面10" through (0, 0, 26) normal (0, 0, 1) x (1, 0, 0) in component "LS_RemovableGrate"
sketch "草图10 (5)" plane through (0, 0, 26) normal (0, 0, 1) x (1, 0, 0) in component "LS_RemovableGrate"
  line L0 (60.3, 220) -> (159.7, 220)
  line L1 (159.7, 220) -> (159.7, 224)
  line L2 (159.7, 224) -> (60.3, 224)
  line L3 (60.3, 224) -> (60.3, 220)
  dimension "d956" = 220
  dimension "d957" = 99.4
  dimension "d958" = 4
  constraint horizontal L0
  constraint vertical L1
  constraint horizontal L2
  constraint vertical L3
  measures "d956" vertical distance of origin L0.start
  measures "d957" horizontal distance of L0.start L0.end
  measures "d958" vertical distance of L0.end L1.end
extrude "Drain slot 9''''" cut sketch "草图10 (5)" along normal blind 4 bodies 10 in component "LS_RemovableGrate"
ref_plane "工作平面11" through (0, 0, 26) normal (0, 0, 1) x (1, 0, 0) in component "LS_RemovableGrate"
sketch "草图11 (5)" plane through (0, 0, 26) normal (0, 0, 1) x (1, 0, 0) in component "LS_RemovableGrate"
  line L0 (60.3, 210) -> (159.7, 210)
  line L1 (159.7, 210) -> (159.7, 214)
  line L2 (159.7, 214) -> (60.3, 214)
  line L3 (60.3, 214) -> (60.3, 210)
  dimension "d964" = 210
  dimension "d965" = 99.4
  dimension "d966" = 4
  constraint horizontal L0
  constraint vertical L1
  constraint horizontal L2
  constraint vertical L3
  measures "d964" vertical distance of origin L0.start
  measures "d965" horizontal distance of L0.start L0.end
  measures "d966" vertical distance of L0.end L1.end
extrude "Drain slot 10''''" cut sketch "草图11 (5)" along normal blind 4 bodies 10 in component "LS_RemovableGrate"
ref_plane "工作平面12" through (0, 0, 26) normal (0, 0, 1) x (1, 0, 0) in component "LS_RemovableGrate"
sketch "草图12 (5)" plane through (0, 0, 26) normal (0, 0, 1) x (1, 0, 0) in component "LS_RemovableGrate"
  line L0 (60.3, 200) -> (159.7, 200)
  line L1 (159.7, 200) -> (159.7, 204)
  line L2 (159.7, 204) -> (60.3, 204)
  line L3 (60.3, 204) -> (60.3, 200)
  dimension "d972" = 200
  dimension "d973" = 99.4
  dimension "d974" = 4
  constraint horizontal L0
  constraint vertical L1
  constraint horizontal L2
  constraint vertical L3
  measures "d972" vertical distance of origin L0.start
  measures "d973" horizontal distance of L0.start L0.end
  measures "d974" vertical distance of L0.end L1.end
extrude "Drain slot 11''''" cut sketch "草图12 (5)" along normal blind 4 bodies 10 in component "LS_RemovableGrate"
ref_plane "工作平面13" through (0, 0, 26) normal (0, 0, 1) x (1, 0, 0) in component "LS_RemovableGrate"
sketch "草图13 (5)" plane through (0, 0, 26) normal (0, 0, 1) x (1, 0, 0) in component "LS_RemovableGrate"
  line L0 (60.3, 190) -> (159.7, 190)
  line L1 (159.7, 190) -> (159.7, 194)
  line L2 (159.7, 194) -> (60.3, 194)
  line L3 (60.3, 194) -> (60.3, 190)
  dimension "d980" = 190
  dimension "d981" = 99.4
  dimension "d982" = 4
  constraint horizontal L0
  constraint vertical L1
  constraint horizontal L2
  constraint vertical L3
  measures "d980" vertical distance of origin L0.start
  measures "d981" horizontal distance of L0.start L0.end
  measures "d982" vertical distance of L0.end L1.end
extrude "Drain slot 12''" cut sketch "草图13 (5)" along normal blind 4 bodies 10 in component "LS_RemovableGrate"
ref_plane "工作平面14" through (0, 0, 26) normal (0, 0, 1) x (1, 0, 0) in component "LS_RemovableGrate"
sketch "草图14 (3)" plane through (0, 0, 26) normal (0, 0, 1) x (1, 0, 0) in component "LS_RemovableGrate"
  line L0 (60.3, 180) -> (159.7, 180)
  line L1 (159.7, 180) -> (159.7, 184)
  line L2 (159.7, 184) -> (60.3, 184)
  line L3 (60.3, 184) -> (60.3, 180)
  dimension "d988" = 180
  dimension "d989" = 99.4
  dimension "d990" = 4
  constraint horizontal L0
  constraint vertical L1
  constraint horizontal L2
  constraint vertical L3
  measures "d988" vertical distance of origin L0.start
  measures "d989" horizontal distance of L0.start L0.end
  measures "d990" vertical distance of L0.end L1.end
extrude "Drain slot 13''" cut sketch "草图14 (3)" along normal blind 4 bodies 10 in component "LS_RemovableGrate"
ref_plane "工作平面15" through (0, 0, 26) normal (0, 0, 1) x (1, 0, 0) in component "LS_RemovableGrate"
sketch "草图15 (3)" plane through (0, 0, 26) normal (0, 0, 1) x (1, 0, 0) in component "LS_RemovableGrate"
  line L0 (60.3, 170) -> (159.7, 170)
  line L1 (159.7, 170) -> (159.7, 174)
  line L2 (159.7, 174) -> (60.3, 174)
  line L3 (60.3, 174) -> (60.3, 170)
  dimension "d996" = 170
  dimension "d997" = 99.4
  dimension "d998" = 4
  constraint horizontal L0
  constraint vertical L1
  constraint horizontal L2
  constraint vertical L3
  measures "d996" vertical distance of origin L0.start
  measures "d997" horizontal distance of L0.start L0.end
  measures "d998" vertical distance of L0.end L1.end
extrude "Drain slot 14''" cut sketch "草图15 (3)" along normal blind 4 bodies 10 in component "LS_RemovableGrate"
ref_plane "工作平面16" through (0, 0, 26) normal (0, 0, 1) x (1, 0, 0) in component "LS_RemovableGrate"
sketch "草图16 (3)" plane through (0, 0, 26) normal (0, 0, 1) x (1, 0, 0) in component "LS_RemovableGrate"
  line L0 (60.3, 160) -> (159.7, 160)
  line L1 (159.7, 160) -> (159.7, 164)
  line L2 (159.7, 164) -> (60.3, 164)
  line L3 (60.3, 164) -> (60.3, 160)
  dimension "d1004" = 160
  dimension "d1005" = 99.4
  dimension "d1006" = 4
  constraint horizontal L0
  constraint vertical L1
  constraint horizontal L2
  constraint vertical L3
  measures "d1004" vertical distance of origin L0.start
  measures "d1005" horizontal distance of L0.start L0.end
  measures "d1006" vertical distance of L0.end L1.end
extrude "Drain slot 15''" cut sketch "草图16 (3)" along normal blind 4 bodies 10 in component "LS_RemovableGrate"
ref_plane "工作平面17" through (0, 0, 26) normal (0, 0, 1) x (1, 0, 0) in component "LS_RemovableGrate"
sketch "草图17 (3)" plane through (0, 0, 26) normal (0, 0, 1) x (1, 0, 0) in component "LS_RemovableGrate"
  line L0 (162.7, 224) -> (167.7, 224)
  line L1 (167.7, 224) -> (167.7, 240)
  line L2 (167.7, 240) -> (162.7, 240)
  line L3 (162.7, 240) -> (162.7, 224)
  dimension "d1011" = 162.7
  dimension "d1012" = 224
  dimension "d1013" = 5
  dimension "d1014" = 16
  constraint horizontal L0
  constraint vertical L1
  constraint horizontal L2
  constraint vertical L3
  measures "d1011" horizontal distance of origin L0.start
  measures "d1012" vertical distance of origin L0.start
  measures "d1013" horizontal distance of L0.start L0.end
  measures "d1014" vertical distance of L0.end L1.end